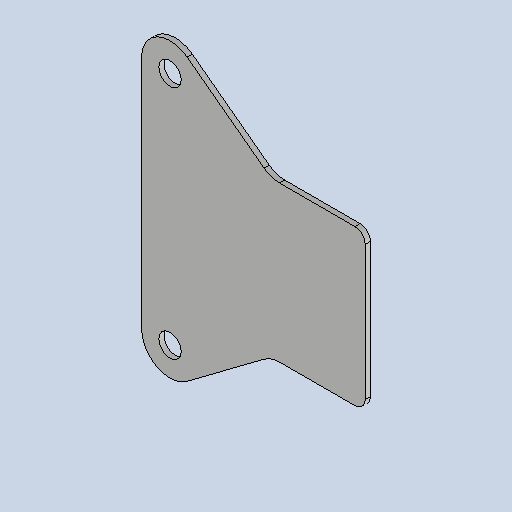
# Autodesk Inventor part: MSC 092 base plate
Saved by Autodesk Inventor 2025 (Build 290162010, 162A)
## iProperties
Created: 2024-07-01
Part Number: MSC 092 base plate
Material: Stainless Steel
Document SubType Name: Sheet Metal
Designer: admin
Density: 8 g/cm^3
Sheet Metal Rule: AISI304 2mm Die16
Appearance: Default
Stock Number: МОО 092 базовая пластина
Author: pokla
Autodesk Inventor part; units mm, degrees
ref_plane "YZ Plane" through (0, 0, 0) normal (1, 0, 0) x (0, 1, 0)
ref_plane "XZ Plane" through (0, 0, 0) normal (0, 1, 0) x (-1, 0, 0)
ref_plane "XY Plane" through (0, 0, 0) normal (0, 0, 1) x (1, 0, 0)
sketch "Sketch1" plane through (0, 0, 0) normal (0, 1, 0) x (-1, 0, 0)
  line L0 (40, 40) -> (-40, 40) construction
  line L1 (-40, 40) -> (-40, -40) construction
  line L2 (-40, -40) -> (40, -40) construction
  line L3 (40, -40) -> (40, 40) construction
  line L4 (-40, 40) -> (40, -40) construction
  line L5 (0, 40) -> (0, -40) construction
  line L6 (84.7843, 0) -> (-45, 0)
  line L7 (-45, -45) -> (-45, 0)
  line L8 (84.7843, 0) -> (84.7843, -68.2843)
  line L9 (4.6857, -45) -> (-45, -45)
  arc A0 (58.3918, -81.4899) -> (84.7843, -68.2843) centre (68.2843, -68.2843) ccw
  circle A1 centre (68.2843, -68.2843) radius 6.5
  line L10 (58.3918, -81.4899) -> (13.6789, -47.9949)
  arc A2 (13.6789, -47.9949) -> (4.6857, -45) centre (4.6857, -60) ccw
  arc A3 (84.7843, -68.2843) -> (58.3918, -81.4899) centre (68.2843, -68.2843) ccw construction
  point P0 (0, 0)
  point P1 (0, 0)
  point P2 (0, 0)
  dimension "d2" = 80
  dimension "d3" = 80
  dimension "d29" = 5
  dimension "d30" = 13
  dimension "d31" = 10
  dimension "d32" = 40
  dimension "d33" = 36.837
  dimension "d34" = 5
  dimension "d35" = 15
  measures "d2" distance of L2.end L1.end
  measures "d3" distance of L1.end L0.end
  measures "d29" distance between parallel lines of L7 L1
  measures "d30" diameter of A1
  measures "d31" radial gap between concentric circles of A0 A1
  measures "d32" distance of L2.end A1.centre
  measures "d33" angle of L2 L10
  measures "d34" distance between parallel lines of L2 L9
  measures "d35" radius of A2
extrude "Plate1" add sketch "Sketch1" along normal blind 3
fillet "Corner Round2" radius 6 1 edges at (45, 1.5, -45)
mirror "Mirror1" about plane through (0, 0, 0) normal (0, 0, 1) of "Plate1", "Corner Round2"
equation "\"d34\" = d29"
equation "\"BendReliefWidth\" = Thickness"
equation "\"BendReliefDepth\" = 0.5 * Thickness"
equation "\"CornerReliefSize\" = 4 * Thickness"
equation "\"MinimumRemnant\" = 2 * Thickness"
equation "\"TransitionRadius\" = BendRadius"
equation "\"JacobiRadiusSize\" = BendRadius"
equation "\"GapSize\" = Thickness"
body "Solid1"
